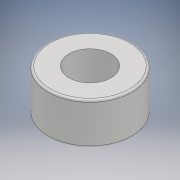
# Autodesk Inventor part: magnes-N35H
Saved by Autodesk Inventor 2017 (Build 210142000, 142)
## iProperties
Created: 2017-03-23
Part Number: magnes-N35H
Material: Magnez
Document SubType Name: Modeling
Designer: Damian
Density: 1.74 g/cm^3
Appearance: Satynowy
Author: Damian
Autodesk Inventor part; units mm, degrees
ref_plane "YZ Plane" through (0, 0, 0) normal (1, 0, 0) x (0, 1, 0)
ref_plane "XZ Plane" through (0, 0, 0) normal (0, 1, 0) x (-1, 0, 0)
ref_plane "XY Plane" through (0, 0, 0) normal (0, 0, 1) x (1, 0, 0)
sketch "Szkic1" plane through (0, 0, 0) normal (0, 0, 1) x (1, 0, 0)
  circle A0 centre (0, 0) radius 2.5
  circle A1 centre (0, 0) radius 5
  dimension "d0" = 5
  dimension "d1" = 10
  constraints: 3 coincident, 2 centre point
  measures "d0" diameter of A0
  measures "d1" diameter of A1
extrude "Wyciągnięcie proste1" add sketch "Szkic1" along normal mid plane 5
fillet "Zaokrąglenie1" radius 0.25 2 edges at (-5, 0, 2.5) (-5, 0, -2.5)
